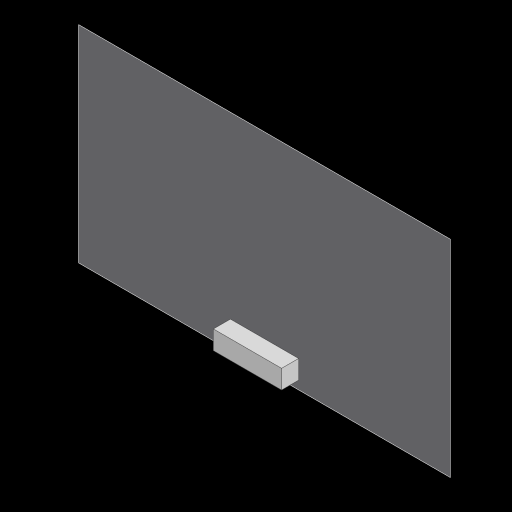
# Autodesk Inventor part: FrontBumper
Saved by Autodesk Inventor 2024 (Build 280153000, 153)
## iProperties
Created: 2026-04-27
Part Number: FrontBumper
Material: Generic
Document SubType Name: Modeling
Designer: Tanner
Density: 1 g/cm^3
Appearance: Default
Author: Tanner
## iProperties of the stored document FrontBumper_3DPrint.ipt
Created: 2026-04-27
Part Number: FrontBumper_3DPrint
Material: Generic
Document SubType Name: Modeling
Designer: Tanner
Density: 1 g/cm^3
Appearance: Default
Author: Tanner
Autodesk Inventor part; units mm, degrees
ref_plane "YZ Plane" through (0, 0, 0) normal (1, 0, 0) x (0, 1, 0)
ref_plane "XZ Plane" through (0, 0, 0) normal (0, 1, 0) x (-1, 0, 0)
ref_plane "XY Plane" through (0, 0, 0) normal (0, 0, 1) x (1, 0, 0)
ref_plane "Work Plane1" through (0, 0, 0) normal (0, 0, 1) x (1, 0, 0)
sketch "Sketch1" plane through (0, 0, 0) normal (0, 0, 1) x (1, 0, 0)
  arc A0 (43.4971, -55) -> (96.8589, 55) centre (0, 34.0439) ccw construction
  line L0 (96.8589, 55) -> (91.8589, 55) construction
  arc A1 (51.9882, -44.5338) -> (91.8589, 55) centre (0, 34.0439) ccw construction
  line L1 (51.9882, -44.5338) -> (-51.9882, -44.5338) construction
  arc A2 (-91.8589, 55) -> (-51.9882, -44.5338) centre (0, 34.0439) ccw construction
  line L2 (-91.8589, 55) -> (-96.8589, 55) construction
  arc A3 (-96.8589, 55) -> (-43.4971, -55) centre (0, 34.0439) ccw construction
  line L3 (-43.4971, -55) -> (43.4971, -55) construction
  circle A4 centre (0, 34.0439) radius 107.6 construction
  arc A5 (43.4971, -55.5561) -> (-43.4971, -55.5561) centre (0, 34.0439) ccw construction
  line L4 (-43.4971, -55.5561) -> (43.4971, -55.5561) construction
  line L5 (-20, -55.5561) -> (20, -55.5561)
  line L6 (20, -55.5561) -> (20, -44.5338)
  line L7 (20, -44.5338) -> (-20, -44.5338)
  line L8 (-20, -44.5338) -> (-20, -55.5561)
  line L9 (20, -44.5338) -> (-20, -55.5561) construction
  line L10 (-20, -44.5338) -> (20, -55.5561) construction
  point P0 (0, 0)
  point P1 (0, -50.045)
  dimension "d0" = 40
  constraints: 12 end point, 2 parallel, 2 point on line, 1 horizontal, 1 midpoint, 1 perpendicular, 1 vertical alignment
  measures "d0" distance between parallel lines of L6 L8
extrude "Extrusion1" add sketch "Sketch1" along normal blind 10
body "Solid1"
